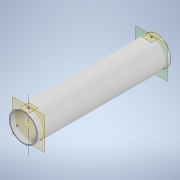
# Autodesk Inventor part: Segment_Engine
Saved by Autodesk Inventor 2020 (Build 240168000, 168)
## iProperties
Created: 2022-01-25
Part Number: Segment_Engine
Material: Generisch
Document SubType Name: Modeling
Designer: sp
Density: 1 g/cm^3
Appearance: Vorgabe
Author: sp
Autodesk Inventor part; units mm, degrees
ref_plane "YZ Plane" through (0, 0, 0) normal (1, 0, 0) x (0, 1, 0)
ref_plane "XZ Plane" through (0, 0, 0) normal (0, 1, 0) x (-1, 0, 0)
sketch "Skizze1" plane through (0, 0, 0) normal (0, 0, 1) x (1, 0, 0)
  circle A0 centre (0, 0) radius 32
  circle A1 centre (0, 0) radius 30
  dimension "d0" = 64
  dimension "d1" = 60
  constraints: 2 centre point, 2 coincident
  measures "d0" diameter of A0
  measures "d1" diameter of A1
extrude "Extrusion1" add sketch "Skizze1" along normal mid plane 300
ref_plane "Arbeitsebene1" through (0, 0, 138.75) normal (0, 0, 1) x (1, 0, 0)
sketch "Skizze2" plane through (0, 0, 138.75) normal (0, 0, 1) x (1, 0, 0)
  line L0 (0, 58.8638) -> (0, -62.7478) construction
  circle A0 centre (0, 0) radius 32 construction
  point P0 (0, 32)
  constraints: 2 end point, 1 point on line, 1 vertical, 1 vertical alignment, 1 other
ref_plane "Arbeitsebene2" through (0, 32, 138.75) normal (0, 1, 0) x (-1, 0, 0)
sketch "Skizze3" plane through (0, 32, 138.75) normal (0, 1, 0) x (-1, 0, 0)
  circle A0 centre (0, 0) radius 1.75
  line L0 (-44.8, 0) -> (44.8, 0) projected
  point P0 (0, -138.75)
  dimension "d5" = 3.5
  constraints: 1 centre point, 1 midpoint
  measures "d5" diameter of A0
extrude "Extrusion2" cut sketch "Skizze3" against normal blind 10
pattern_circular "Runde Anordnung1" count 3 over 360 about axis through (0, 0, -10) along (0, 0, 1) of "Extrusion2"
mirror "Spiegeln1" about plane through (0, 0, 0) normal (0, 0, 1) of "Extrusion2", "Runde Anordnung1"
ref_plane "Arbeitsebene3" through (0, 0, -138.75) normal (0, 0, 1) x (1, 0, 0)
ref_plane "Arbeitsebene4" through (0, 32, -138.75) normal (0, -1, 0) x (-1, 0, 0)
